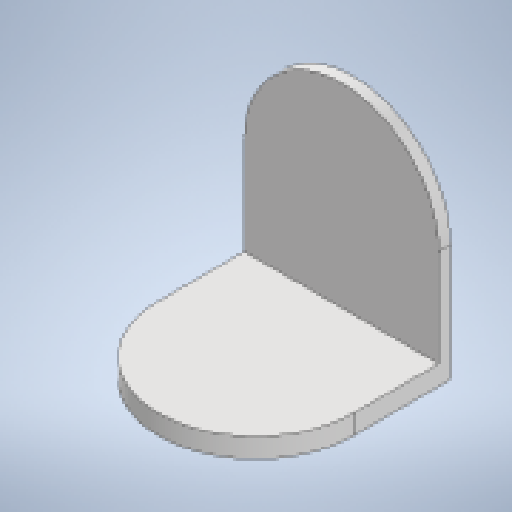
# Autodesk Inventor part: Base_1
Saved by Autodesk Inventor 2023 (Build 270158000, 158)
## iProperties
Created: 2022-04-08
Part Number: Base_1
Material: 一般
Document SubType Name: Modeling
Designer: device
Density: 1 g/cm^3
Appearance: 預設
Author: device
Autodesk Inventor part; units mm, degrees
ref_plane "YZ Plane" through (0, 0, 0) normal (1, 0, 0) x (0, 1, 0)
ref_plane "XZ Plane" through (0, 0, 0) normal (0, 1, 0) x (-1, 0, 0)
ref_plane "XY Plane" through (0, 0, 0) normal (0, 0, 1) x (1, 0, 0)
sketch "草圖1" plane through (0, 0, 0) normal (0, 1, 0) x (-1, 0, 0)
  circle A0 centre (0, 0) radius 25
  line L0 (25, 0) -> (-25, 0)
  line L1 (-25, 0) -> (-25, -25)
  line L2 (-25, -25) -> (25, -25)
  line L3 (25, -25) -> (25, 0)
  dimension "d0" = 50
  constraints: 8 end point, 2 parallel, 1 coincident, 1 horizontal, 1 perpendicular, 3 other
extrude "擠出1" add sketch "草圖1" along normal mid plane 3
sketch "草圖2" plane through (0, 1.5, 0) normal (0, 1, 0) x (1, 0, 0)
  line L0 (-25, 25) -> (-25, 0) projected
  line L1 (25, 0) -> (25, 25) projected
  line L2 (-25, 25) -> (25, 25)
  line L3 (25, 25) -> (25, 22)
  line L4 (25, 22) -> (-25, 22)
  line L5 (-25, 22) -> (-25, 25)
  point P0 (0, 0)
  dimension "d3" = 3
  constraints: 8 end point, 2 parallel, 1 horizontal, 1 perpendicular, 1 point on line
  measures "d3" distance of L2.end L3.end
extrude "擠出2" add sketch "草圖2" along normal blind 50
sketch "草圖3" plane through (-25, 1.5, -22) normal (0, 0, 1) x (1, 0, 0)
  circle A0 centre (25, 25) radius 25
  line L0 (0, 50) -> (50, 50) projected
  line L1 (50, 0) -> (50, 50) projected
  line L2 (50, 0) -> (0, 0) projected
  line L3 (50, 0) -> (50, 50) projected
  line L4 (0, 50) -> (50, 50) projected
  line L5 (0, 0) -> (0, 50) projected
  point P0 (25, -1.5)
  point P1 (25, 50)
  point P2 (0, 25)
  point P3 (50, 25)
  constraints: 1 horizontal, 1 midpoint, 1 vertical, 3 other
extrude "擠出3" cut sketch "草圖3" against normal up to surface (3 mm away) contours A0 L0 L1 | A0 L5 L0
